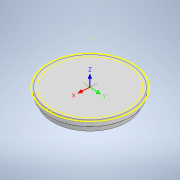
# Autodesk Inventor part: Head_V6_modified
Saved by Autodesk Inventor 2020 (Build 240168000, 168)
## iProperties
Created: 2021-06-29
Part Number: Head_V6_modified
Material: Generic
Document SubType Name: Modeling
Designer: jeten
Density: 1 g/cm^3
Appearance: Default
Author: jeten
## iProperties of the stored document _3DPrint.ipt
Created: 2021-06-29
Part Number: _3DPrint
Material: Generic
Document SubType Name: Modeling
Designer: jeten
Density: 1 g/cm^3
Appearance: Default
Author: jeten
Autodesk Inventor part; units mm, degrees
ref_plane "YZ Plane" through (0, 0, 0) normal (1, 0, 0) x (0, 1, 0)
ref_plane "XZ Plane" through (0, 0, 0) normal (0, 1, 0) x (-1, 0, 0)
ref_plane "XY Plane" through (0, 0, 0) normal (0, 0, 1) x (1, 0, 0)
sketch "Sketch1" plane through (48.8758, 103.3243, 1.0364) normal (0, 1, 0) x (-1, 0, 0)
  circle A0 centre (-11.1015, 58.9409) radius 59.9773 projected
  line L0 (-7.4528, 118.1058) -> (-7.4529, 112.0932) projected
  circle A1 centre (-11.101, 58.953) radius 53.2652 projected
  circle A2 centre (-11.1016, 58.9392) radius 59.279 projected
  line L1 (-13.4524, 112.1664) -> (-13.4524, 118.1716) projected
  point P0 (48.8758, -1.0364)
  constraints: 2 other
sketch "Sketch2" plane through (59.9773, 103.3243, 59.9773) normal (0, 1, 0) x (-0.0684835, 0, 0.9976522)
  line L0 (17.4535, -14.1995) -> (19.2244, -11.6906)
  line L1 (-19.2244, -11.6906) -> (-20.6373, -8.964)
  line L2 (1.5354, 22.4475) -> (4.5778, 22.0294)
  ellipse E0 centre (-15.8457, 0.0738) end of major axis (-15.8594, -3.2475) minor radius 3.2638
  ellipse E1 centre (9.6568, 14.831) end of major axis (6.8501, 16.6607) minor radius 3.2778
  ellipse E2 centre (9.8276, -14.769) end of major axis (7.0654, -16.6064) minor radius 3.2452
  circle A0 centre (0, 0) radius 22.4475
  circle A1 centre (0, 0) radius 17.7399
  ellipse E3 centre (17.7399, 0) end of major axis (14.9777, -1.8375) minor radius 3.2452
  point P0 (0, 0)
  constraints: 6 end point, 3 tangent, 2 centre point, 2 point on circle, 1 coincident, 8 other
sketch "HeadSlice" plane through (59.9773, 103.3243, 59.9773) normal (-0.0684835, 0, 0.9976522) x (0.9976522, 0, 0.0684835)
  line L0 (-59.9381, -8.5562) -> (-59.9741, -8.5562) projected
  line L1 (-59.8803, -8.5562) -> (-59.9741, -8.5562) projected
  line L2 (-59.9741, -8.5562) -> (-59.9381, -8.5562) projected
  line L3 (-55.6562, -17.256) -> (-55.6559, -17.256) projected
  line L4 (-55.5803, -17.256) -> (-55.6689, -17.256) projected
  line L5 (-55.6639, -17.256) -> (19.7894, -17.256) projected
  line L6 (20.141, -16.8756) -> (-55.0671, -16.8756) projected
  line L7 (-27.4611, -4.5822) -> (-27.4997, -4.5822) projected
  line L8 (-27.4693, -4.5822) -> (-27.4997, -4.5822) projected
  line L9 (-17.5004, -2.3292) -> (-17.4829, -2.3292) projected
  line L10 (0, -20.7072) -> (0, 3.4512) projected
  line L11 (-52.7836, -17.256) -> (-52.1868, -16.8756)
  line L12 (-56.3971, -8.2984) -> (-56.3971, -1.1)
  line L13 (-27.4969, -1.0968) -> (-27.4693, -4.5822)
  line L14 (-27.4693, -4.5822) -> (-17.4829, -2.3292)
  line L15 (-10.4205, -0.7359) -> (0, -0.7)
  line L16 (-56.96, -8.6389) -> (-52.7836, -17.256)
  line L17 (-27.8969, -0.7) -> (-55.9971, -0.7)
  line L18 (-56.3554, -8.4762) -> (-52.1868, -16.8756)
  line L19 (-57, -8.4644) -> (-57, 0)
  line L20 (-57, 0) -> (2.8803, 0)
  line L21 (0, -0.7) -> (0, 0)
  arc A0 (-55.9971, -0.7) -> (-56.3971, -1.1) centre (-55.9971, -1.1) ccw
  arc A1 (-27.4969, -1.0968) -> (-27.8969, -0.7) centre (-27.8969, -1.1) ccw
  arc A2 (-56.3971, -8.2984) -> (-56.3554, -8.4762) centre (-55.9971, -8.2984) ccw
  arc A3 (-57, -8.4644) -> (-56.96, -8.6389) centre (-56.6, -8.4644) ccw
  line L22 (-57, 0) -> (0, 0)
  line L23 (-17.4829, -2.3292) -> (-10.4205, -0.7359)
  line L24 (-57, 0) -> (0, 0)
  point P0 (-59.2773, -0.7)
  point P1 (-27.5, -0.7)
  point P2 (-52.968, -16.8756)
  point P3 (-52.1868, -16.8756)
  dimension "d6" = 0.4
  constraints: 28 end point, 8 point on circle, 7 tangent, 4 centre point, 4 point on line, 3 collinear, 3 equal radius, 1 vertical
  measures "d6" radius of A0
revolve "Revolution1" add sketch "HeadSlice" angle 360 about axis through (59.9773, 93.3243, 59.9773) along (0, 1, 0) contours L6 L16 A3 L19 L20 L10 L15 L23 L14 L7 L13 A1 L17 A0 L12 A2 L18
extrude "Extrusion1" [suppressed]
body "Solid1"
